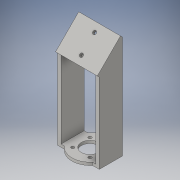
# Autodesk Inventor part: MotorMount
Saved by Autodesk Inventor 2016 (Build 200138000, 138)
## iProperties
Created: 2015-09-29
Part Number: MotorMount
Material: Generic
Document SubType Name: Modeling
Designer: Mack
Density: 1 g/cm^3
Appearance: Default
Author: Mack
Autodesk Inventor part; units mm, degrees
ref_plane "YZ Plane" through (0, 0, 0) normal (1, 0, 0) x (0, 1, 0)
ref_plane "XZ Plane" through (0, 0, 0) normal (0, 1, 0) x (-1, 0, 0)
ref_plane "XY Plane" through (0, 0, 0) normal (0, 0, 1) x (1, 0, 0)
sketch "Sketch1" plane through (0, 0, 0) normal (0, 1, 0) x (-1, 0, 0)
  circle A0 centre (0, 0) radius 26
  circle A1 centre (0, 0) radius 12.5
  dimension "d0" = 52
  dimension "d15" = 25
  constraints: 2 centre point, 2 coincident
  measures "d0" diameter of A0
  measures "d15" diameter of A1
extrude "Extrusion1" add sketch "Sketch1" along normal blind 4 contours A0 | A1
sketch "Sketch2" plane through (0, 4, 0) normal (0, 1, 0) x (1, 0, 0)
  line L0 (-30, 16.6132) -> (-20, 16.6132)
  line L1 (-20, -16.6132) -> (-30, -16.6132)
  line L2 (-30, -16.6132) -> (-30, 16.6132)
  line L3 (0, 41.9312) -> (0, 29.2053)
  line L4 (30, 16.6132) -> (20, 16.6132)
  line L5 (20, -16.6132) -> (30, -16.6132)
  line L6 (30, -16.6132) -> (30, 16.6132)
  line L7 (-20, 16.6132) -> (-20, 11.3578)
  line L8 (-20, -11.3578) -> (-20, -16.6132)
  line L9 (20, 16.6132) -> (20, 11.3578)
  line L10 (20, -11.3578) -> (20, -16.6132)
  arc A0 (-20, 11.3578) -> (-20, -11.3578) centre (0, 0) ccw
  arc A1 (20, -11.3578) -> (20, 11.3578) centre (0, 0) ccw
  constraints: 22 end point, 4 point on circle, 4 symmetric about line, 3 parallel, 2 centre point, 2 perpendicular, 1 horizontal, 1 vertical
extrude "Extrusion2" add sketch "Sketch2" against normal blind 4
sketch "Sketch3" plane through (0, 4, 0) normal (0, 1, 0) x (1, 0, 0)
  line L0 (-30, 16.6132) -> (-20, 16.6132) projected
  line L1 (-20, -16.6132) -> (-30, -16.6132) projected
  line L2 (-30, 16.6132) -> (-25, 16.6132)
  line L3 (-25, 16.6132) -> (-25, -16.6132)
  line L4 (-25, -16.6132) -> (-30, -16.6132)
  line L5 (-30, -16.6132) -> (-30, 16.6132)
  line L6 (20, 16.6132) -> (30, 16.6132) projected
  line L7 (30, -16.6132) -> (20, -16.6132) projected
  line L8 (30, 16.6132) -> (25, 16.6132)
  line L9 (25, 16.6132) -> (25, -16.6132)
  line L10 (25, -16.6132) -> (30, -16.6132)
  line L11 (30, -16.6132) -> (30, 16.6132)
  point P0 (0, 0)
  dimension "d12" = 5
  constraints: 16 end point, 4 parallel, 2 horizontal, 2 midpoint, 2 perpendicular
  measures "d12" distance between parallel lines of L5 L3
extrude "Extrusion3" add sketch "Sketch3" along normal blind 144
sketch "Sketch4" plane through (0, 4, 0) normal (0, 1, 0) x (1, 0, 0)
  circle A0 centre (0, 0) radius 12.5
  dimension "d16" = 25
  constraints: 1 centre point, 1 coincident
  measures "d16" diameter of A0
extrude "Extrusion4" cut sketch "Sketch4" against normal blind 4
sketch "Sketch5" plane through (0, 0, 0) normal (0, -1, 0) x (1, 0, 0)
  point P0 (0, 0)
  point P1 (-12.3744, 12.3744)
  point P2 (12.3744, 12.3744)
  point P3 (12.3744, -12.3744)
  point P4 (-12.3744, -12.3744)
  dimension "d19" = 12.3744
  dimension "d20" = 12.3744
  dimension "d23" = 360
  constraints: 5 other
  measures "d19" horizontal distance of point (0, 0) point (-12.374, 12.374)
  measures "d20" horizontal distance of point (0, 0) point (-12.374, 12.374)
hole "Hole1" at (-12.3744, 0, 12.3744) at (12.3744, 0, 12.3744) at (12.3744, 0, -12.3744) at (-12.3744, 0, -12.3744) direction (0, 1, 0) diameter 4.5 end through all
chamfer "Chamfer1" distance 33.226 angle 45 2 edges at (27.5, 148, 16.6132) (-27.5, 148, 16.6132)
sketch "Sketch6" plane through (-30, 148, -16.6128) normal (0, 0.7071, 0.7071) x (1, 0, 0)
  line L0 (0, -104.6515) -> (0, 0.0004) projected
  line L1 (55, -46.9887) -> (60, -46.9887) projected
  line L2 (0, 0.0004) -> (60, 0.0004)
  line L3 (60, 0.0004) -> (60, -46.9887)
  line L4 (60, -46.9887) -> (0, -46.9887)
  line L5 (0, -46.9887) -> (0, 0.0004)
  point P0 (30, -116.3988)
  constraints: 8 end point, 2 parallel, 1 horizontal, 1 perpendicular
extrude "Extrusion5" add sketch "Sketch6" along normal blind 4
sketch "Sketch7" plane through (-30, 150.8284, -13.7843) normal (0, 0.7071, 0.7071) x (1, 0, 0)
  line L0 (0, 0.0004) -> (0, -46.9887) projected
  line L1 (60, -46.9887) -> (60, 0.0004) projected
  line L2 (60, 0.0004) -> (0, 0.0004) projected
  line L3 (0, -46.9887) -> (60, -46.9887) projected
  point P0 (30, -116.3988)
  point P1 (30, -10.1596)
  point P2 (30, -36.8287)
  dimension "d37" = 60
  dimension "d38" = 30
  dimension "d39" = 10.16
  dimension "d40" = 10.16
  measures "d37" distance between parallel lines of L0 L1
  measures "d38" distance from line of point (30, -10.16) L1
  measures "d39" distance from line of L2 point (30, -10.16)
  measures "d40" distance from line of L3 point (30, -36.829)
hole "Hole2" at (0, 143.6445, -6.6004) at (0, 124.7866, 12.2575) direction (0, -0.7071, -0.7071) diameter 5 end through all
equation "\"d20\" = d19"
equation "\"d38\" = 0.5 * d37"
body "Solid1"
